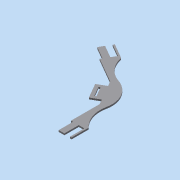
# Autodesk Inventor part: brazos
Saved by Autodesk Inventor 2015 (Build 190159000, 159)
## iProperties
Created: 2017-10-02
Part Number: brazos
Material: Generic
Document SubType Name: Modeling
Designer: macbook
Density: 1 g/cm^3
Appearance: Default
Author: macbook
Autodesk Inventor part; units mm, degrees
ref_plane "YZ Plane" through (0, 0, 0) normal (1, 0, 0) x (0, 1, 0)
ref_plane "XZ Plane" through (0, 0, 0) normal (0, 1, 0) x (-1, 0, 0)
ref_plane "XY Plane" through (0, 0, 0) normal (0, 0, 1) x (1, 0, 0)
sketch "Sketch1" plane through (0, 0, 0) normal (0, 0, 1) x (1, 0, 0)
  arc A0 (20, 100) -> (52, 10) centre (115.8042, 83.3748) ccw
  line L0 (-10, 117.3205) -> (-38.5788, 100.8205)
  line L1 (-38.5788, 100.8205) -> (-68.5788, 152.782)
  line L2 (-68.5788, 152.782) -> (-40, 169.282)
  line L3 (-29.2894, 117.7308) -> (-34.0526, 114.9808)
  line L4 (-34.0526, 114.9808) -> (-54.0526, 149.6218)
  line L5 (-54.0526, 149.6218) -> (-49.2894, 152.3718)
  line L6 (-49.2894, 152.3718) -> (-29.2894, 117.7308)
  line L7 (46.5, 0) -> (46.5, -50)
  line L8 (46.5, -50) -> (52, -50)
  line L9 (52, -50) -> (52, 0)
  line L10 (-136.6025, 236.6025) -> (-50, 186.6025)
  arc A1 (-101.9423, 276.6359) -> (-40, 203.923) centre (-6.4957, 295.2045) ccw
  line L11 (-136.6025, 236.6025) -> (-50, 186.6025)
  arc A2 (20, 100) -> (-40, 203.923) centre (-65.07, 120.1668) ccw
  line L12 (-10, 117.3205) -> (0, 100)
  line L13 (-40, 169.282) -> (-50, 186.6025)
  line L14 (0, 100) -> (0, 0)
  line L15 (52, 10) -> (52, 0)
  line L16 (-110.6025, 281.6359) -> (-101.9423, 276.6359)
  line L17 (46.5, 0) -> (27.071, 0)
  line L18 (27.071, 0) -> (27.071, -50)
  line L19 (27.071, -50) -> (7.071, -50)
  line L20 (7.071, -50) -> (7.071, 0)
  line L21 (7.071, 0) -> (0, 0)
  line L22 (-136.6025, 236.6025) -> (-133.067, 242.7262)
  line L23 (-136.6025, 236.6025) -> (-129.5315, 236.6025) construction
  line L24 (-133.067, 242.7262) -> (-176.3683, 267.7262)
  line L25 (-176.3683, 267.7262) -> (-166.3683, 285.0467)
  line L26 (-166.3683, 285.0467) -> (-123.067, 260.0467)
  line L27 (-123.067, 260.0467) -> (-113.3525, 276.8727)
  line L28 (-113.3525, 276.8727) -> (-156.6538, 301.8727)
  line L29 (-156.6538, 301.8727) -> (-153.9038, 306.6359)
  line L30 (-153.9038, 306.6359) -> (-110.6025, 281.6359)
  dimension "d9" = 33
  dimension "d10" = 60
  dimension "d11" = 5.5
  dimension "d12" = 40
  dimension "d13" = 52
  dimension "d14" = 100
  dimension "d18" = 5.5
  dimension "d28" = 19.429
  dimension "d29" = 20
  dimension "d30" = 50
  dimension "d31" = 50
  dimension "d32" = 7.071
  dimension "d33" = 7.071
  dimension "d34" = 60
  dimension "d35" = 50
  dimension "d36" = 90
  dimension "d37" = 20
  dimension "d38" = 90
  dimension "d39" = 19.429
  dimension "d40" = 5.5
  constraints: 62 end point, 10 perpendicular, 6 equal length, 6 point on circle, 3 centre point, 3 horizontal, 3 point on line, 2 vertical
  measures "d9" distance of L1.end L2.end
  measures "d10" distance of L0.end L1.end
  measures "d11" distance of L4.end L5.end
  measures "d12" distance of L3.end L4.end
  measures "d13" distance of L14.end L9.end
  measures "d14" distance of L14.end L12.end
  measures "d18" distance of L8.end L7.end
  measures "d28" distance of L7.start L17.end
  measures "d29" distance of L18.end L19.end
  measures "d30" distance between parallel lines of L8 L17
  measures "d31" distance between parallel lines of L21 L19
  measures "d32" distance between parallel lines of L14 L20
  measures "d33" distance of L11.start L22.end
  measures "d34" angle of L23 L22
  measures "d35" distance of L22.end L24.end
  measures "d36" angle of L24 L22
  measures "d37" distance of L24.end L25.end
  measures "d38" angle of L25 L26
  measures "d39" distance of L26.end L27.end
  measures "d40" distance of L28.end L29.end
extrude "Extrusion2" add sketch "Sketch1" along normal blind 5.5
body "Solid2"
